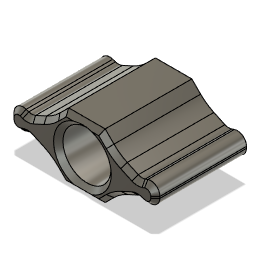
3-16OD tube clincher for 3mm pump v2 (Autodesk Fusion 360 design; units mm, degrees)
Autodesk Fusion 360 part; units mm, degrees
sketch "Sketch1" plane through (0, 0, 0) normal (0, 0, 1) x (1, 0, 0)
  circle A0 centre (0, 0) radius 2.295
  circle A1 centre (0, 0) radius 1.475
  line L0 (8, -3.5) -> (-8, -3.5)
  line L1 (-8, -3.5) -> (-8, 3.5)
  line L2 (-8, 3.5) -> (8, 3.5)
  line L3 (8, 3.5) -> (8, -3.5)
  line L4 (8, -3.5) -> (-8, 3.5) construction
  line L5 (-8, -3.5) -> (8, 3.5) construction
  dimension "d1" = 4.7625
  dimension "d2" = 2.95
  dimension "d3" = 0.82
  dimension "d4" = 16
  dimension "d5" = 7
  constraint coincident A0.centre A1.centre
  constraint concentric A0 A1
  constraint horizontal L0
  constraint perpendicular L0 L1
  constraint parallel L0 L2
  constraint parallel L1 L3
  constraint coincident L4 A0.centre
  constraint coincident L5 A0.centre
  measures "d2" diameter of A1
  measures "d3" distance of A0 A1
  measures "d4" distance of L0.start L0.end
  measures "d5" distance of L0.start L2.end
extrude "Extrude1" add sketch "Sketch1" along normal blind 10 contours L0 L1 L2 L3
ref_plane "WorkPlane1" through (0, 0, 3) normal (0, 0, 1) x (1, 0, 0)
sketch "Sketch2" plane through (0, 0, 10) normal (0, 0, 1) x (1, 0, 0)
  circle A0 centre (0, 0) radius 2.295
  line L0 (8, 3.5) -> (-8, 3.5)
  line L1 (-8, 3.5) -> (-8, -3.5)
  line L2 (-8, -3.5) -> (8, -3.5)
  line L3 (8, -3.5) -> (8, 3.5)
  line L4 (-2, -3.5) -> (-3.6, -1.9)
  line L5 (-8, -1.5) -> (-8, 0)
  line L6 (-8, 0) -> (0, 0)
  line L7 (0, 0) -> (0, -3.5)
  line L8 (-2, -3.5) -> (0, -3.5)
  line L9 (-8, -1.5) -> (-6, -0.8)
  line L10 (-6, -0.8) -> (-3.6, -1.9)
  dimension "d10" = 2
  dimension "d11" = 1.6
  dimension "d17" = 1.6
  dimension "d18" = 3
  dimension "d19" = 2
  dimension "d20" = 1.6
  constraint coincident L2 L4.start
  constraint coincident L1 L5.start
  constraint coincident L1 L5.end
  constraint midpoint L1 L5.end
  constraint coincident A0.centre L6.end
  constraint midpoint L2 L7.end
  measures "d10" distance of L4.start L7.end
  measures "d11" horizontal distance of L4.start L4.end
  measures "d19" horizontal distance of L5.start L9.end
  measures "d20" vertical distance of L4.start L4.end
extrude "Extrude2" cut sketch "Sketch2" against normal through all contours L1 L2 L4 L9 L10
mirror "Mirror1" about plane through (0, 0, 0) normal (0, 1, 0) of "Extrude2"
mirror "Mirror2" about plane through (0, 0, 0) normal (1, 0, 0) of "Extrude2", "Mirror1"
fillet "Fillet1" radius 1 8 edges at (-8, -1.5, 5) (-6, -0.8, 5) (-8, 1.5, 5) (-6, 0.8, 5) (6, -0.8, 5) (6, 0.8, 5) (8, 1.5, 5) (8, -1.5, 5)
fillet "Fillet1" radius 5 4 edges at (-3.6, -1.9, 5) (-3.6, 1.9, 5) (3.6, -1.9, 5) (3.6, 1.9, 5)
split_face "SplitFace1" 1 faces at (2.2921, -0.1144, 6.6667) by plane through (0, 0, 3) normal (0, 0, 1)
draft "Draft1" angle 3 neutral plane through (0, 0, 3) pull (0, 0, 1) 1 faces at (2.2836, 0.2285, 5.3333)
chamfer "Chamfer1" distance 0.5 angle 45 1 edges at (-2.4817, 0.9626, 10)
chamfer "Chamfer1" distance 0.5 angle 45 28 edges at (3.6457, -1.9658, 10) (2.4823, -3.0177, 10) (2.4823, 3.0177, 10) (3.6457, 1.9658, 10) (5.0252, 1.2468, 10) (6.0036, 0.8781, 10) (6.5251, 0.9838, 10) (7.5786, 0.9061, 10) (8, 0, 10) (7.5786, -0.9061, 10) (6.5251, -0.9838, 10) (6.0036, -0.8781, 10) (5.0252, -1.2468, 10) (0, -3.5, 10) (-3.6457, -1.9658, 10) (-5.0252, -1.2468, 10) (-6.0036, -0.8781, 10) (-6.5251, -0.9838, 10) (-7.5786, -0.9061, 10) (-8, 0, 10) (-7.5786, 0.9061, 10) (-6.5251, 0.9838, 10) (-6.0036, 0.8781, 10) (-5.0252, 1.2468, 10) (-3.6457, 1.9658, 10) (-2.4823, 3.0177, 10) (-2.4823, -3.0177, 10) (0, 3.5, 10)
equation "d1 = 3 / 16 * in"
